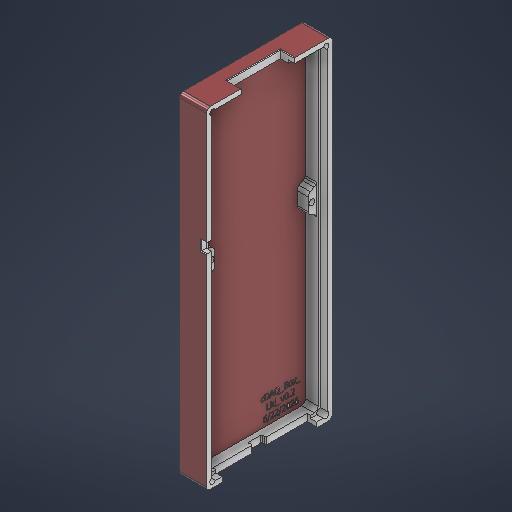
# Autodesk Inventor part: cDAQ_Box_Lid_v0.2
Saved by Autodesk Inventor 2027 (Build 310192000, 192)
## iProperties
Created: 2026-05-08
Part Number: cDAQ_Box_Lid_v0.2
Material: Generic
Document SubType Name: Modeling
Designer: giese
Density: 1 g/cm^3
Appearance: Default
Author: giese
Autodesk Inventor part; units mm, degrees
(part 1 of 2)
ref_plane "YZ Plane" through (0, 0, 0) normal (1, 0, 0) x (0, 1, 0)
ref_plane "XZ Plane" through (0, 0, 0) normal (0, 1, 0) x (-1, 0, 0)
ref_plane "XY Plane" through (0, 0, 0) normal (0, 0, 1) x (1, 0, 0)
sketch "Sketch1" plane through (0, 0, 0) normal (1, 0, 0) x (0, 1, 0)
  line L0 (50.7569, 48.4212) -> (-216.9591, 48.4212)
  line L1 (-216.9591, 48.4212) -> (-216.9591, -53.1788)
  line L2 (-216.9591, -53.1788) -> (50.7569, -53.1788)
  line L3 (50.7569, -53.1788) -> (50.7569, 48.4212)
  point P0 (0, 0)
  dimension "d0" = 101.6
  dimension "d1" = 267.716
  constraints: 8 end point, 2 parallel, 1 horizontal, 1 perpendicular
  measures "d0" distance of L2.end L0.start
  measures "d1" distance of L0.start L0.end
extrude "Extrusion1" add sketch "Sketch1" along normal blind 21.59
sketch "Sketch2" plane through (21.59, 0, 0) normal (1, 0, 0) x (0, 0, -1)
  line L0 (-42.0712, 44.4069) -> (46.8288, 44.4069)
  line L1 (46.8288, 44.4069) -> (46.8288, -210.6091)
  line L2 (46.8288, -210.6091) -> (-42.0712, -210.6091)
  line L3 (-42.0712, -210.6091) -> (-42.0712, 44.4069)
  line L4 (-48.4212, 50.7569) -> (-48.4212, -216.9591) projected
  line L5 (-48.4212, -216.9591) -> (53.1788, -216.9591) projected
  point P0 (0, 0)
  dimension "d4" = 88.9
  dimension "d5" = 255.016
  dimension "d6" = 6.35
  dimension "d7" = 6.35
  constraints: 8 end point, 2 parallel, 1 horizontal, 1 perpendicular
  measures "d4" distance of L0.start L0.end
  measures "d5" distance of L0.end L1.end
  measures "d6" distance between parallel lines of L4 L3
  measures "d7" distance between parallel lines of L5 L2
extrude "Extrusion2" cut sketch "Sketch2" against normal blind 15.24
sketch "Sketch3" plane through (0, 0, 0) normal (-1, 0, 0) x (0, 0, 1)
  circle A0 centre (-30.3188, 7.3229) radius 2
  line L0 (-53.1788, -216.9591) -> (-53.1788, 50.7569) projected
  line L1 (-53.1788, 50.7569) -> (48.4212, 50.7569) projected
  circle A1 centre (-11.82, 7.3229) radius 2
  circle A2 centre (6.6789, 7.3229) radius 2
  point P0 (0, 0)
  dimension "d10" = 22.86
  dimension "d11" = 43.434
  dimension "d12" = 43.434
  dimension "d13" = 18.4988
  dimension "d14" = 4
  dimension "d15" = 4
  dimension "d16" = 43.434
  dimension "d17" = 18.4988
  dimension "d18" = 36.9976
  dimension "d21" = 4
  constraints: 3 centre point
  measures "d10" distance from line of L0 A0.centre
  measures "d11" distance from line of L1 A0.centre
  measures "d12" distance from line of L1 A1.centre
  measures "d13" distance of A0.centre A1.centre
  measures "d14" diameter of A1
  measures "d15" diameter of A2
  measures "d16" distance from line of L1 A2.centre
  measures "d17" distance of A1.centre A2.centre
  measures "d18" distance of A0.centre A2.centre
  measures "d21" diameter of A0
extrude "Extrusion3" [suppressed]
sketch "Sketch6" plane through (0, 50.7569, 48.4212) normal (0, 1, 0) x (1, 0, 0)
  line L0 (21.59, 6.35) -> (21.59, 95.25) projected
  line L1 (10.16, 27.94) -> (21.59, 27.94)
  line L2 (21.59, 27.94) -> (21.59, 71.12)
  line L3 (21.59, 71.12) -> (10.16, 71.12)
  line L4 (10.16, 71.12) -> (10.16, 27.94)
  line L5 (0, 101.6) -> (21.59, 101.6) projected
  point P0 (0, 48.4212)
  point P1 (15.875, 71.12)
  point P2 (15.875, 27.94)
  dimension "d30" = 11.43
  dimension "d31" = 43.18
  dimension "d32" = 30.48
  constraints: 8 end point, 2 midpoint, 2 parallel, 1 horizontal, 1 perpendicular, 1 point on line
  measures "d30" distance between parallel lines of L0 L4
  measures "d31" distance of point (15.875, 71.12) point (15.875, 27.94)
  measures "d32" distance between parallel lines of L5 L3
extrude "Extrusion5" cut sketch "Sketch6" against normal blind 6.35
fillet "Fillet1" radius 3.175 4 edges at (10.795, 50.7569, -53.1788) (10.795, 50.7569, 48.4212) (10.795, -216.9591, 48.4212) (10.795, -216.9591, -53.1788)
sketch "Sketch7" plane through (21.59, 0, 0) normal (1, 0, 0) x (0, 0, -1)
  line L0 (-42.0712, -210.6091) -> (-42.0712, 44.4069) projected
  line L1 (-42.0712, 44.4069) -> (-42.3252, 44.4069)
  line L2 (-42.3252, 46.6929) -> (-44.2302, 46.6929)
  line L3 (-44.2302, 46.6929) -> (-44.2302, 51.0109)
  line L4 (-42.0712, -190.1621) -> (-42.0712, -210.6091)
  line L5 (46.8288, -210.6091) -> (-42.0712, -210.6091) projected
  line L6 (-40.4202, -212.8951) -> (-44.2302, -212.8951)
  line L7 (-44.2302, -212.8951) -> (-44.2302, -190.1621)
  line L8 (46.8288, 44.4069) -> (46.8288, -210.6091) projected
  line L9 (46.8288, -192.7021) -> (46.8288, -210.6091)
  line L10 (46.8288, -210.6091) -> (43.9078, -210.6091)
  line L11 (46.8288, -210.6091) -> (46.8288, -192.7021)
  line L12 (48.9878, -192.7021) -> (48.9878, -212.8951)
  line L13 (48.9878, -212.8951) -> (43.9078, -212.8951)
  line L14 (-42.0712, 44.4069) -> (46.8288, 44.4069) projected
  line L15 (42.0028, 44.4069) -> (46.8288, 44.4069)
  line L16 (48.9878, 48.4709) -> (48.9878, 46.6929)
  line L17 (48.9878, 46.6929) -> (42.0028, 46.6929)
  line L18 (-42.3252, 46.6929) -> (42.0028, 46.6929)
  line L19 (42.0028, 44.4069) -> (-42.3252, 44.4069)
  line L20 (48.9878, 48.4709) -> (48.9878, -192.7021)
  line L21 (44.2888, -195.2421) -> (44.2888, 44.4069)
  line L22 (43.9078, -210.6091) -> (-40.4202, -210.6091)
  line L23 (-40.4202, -212.8951) -> (43.9078, -212.8951)
  line L24 (-44.2302, -190.1621) -> (-44.2302, 51.0109)
  line L25 (-42.0712, 44.4069) -> (-42.0712, -190.1621)
  point P0 (0, 0)
  point P1 (-42.0712, 51.0109)
  point P2 (-44.2302, 48.9789)
  point P3 (46.8288, 48.4709)
  point P4 (48.9878, 46.6929)
  point P5 (-44.2302, 46.6929)
  dimension "d34" = 2.286
  dimension "d35" = 2.159
  dimension "d38" = 2.159
  dimension "d39" = 2.286
  dimension "d42" = 2.286
  dimension "d43" = 2.159
  dimension "d46" = 2.286
  dimension "d47" = 2.159
  constraints: 44 end point, 9 point on line, 4 parallel, 4 perpendicular, 2 collinear, 2 horizontal, 2 vertical
  measures "d34" distance between parallel lines of L2 L1
  measures "d35" distance between parallel lines of L0 L3
  measures "d38" distance between parallel lines of L7 L0
  measures "d39" distance between parallel lines of L5 L6
  measures "d42" distance between parallel lines of L5 L13
  measures "d43" distance between parallel lines of L8 L12
  measures "d46" distance between parallel lines of L14 L17
  measures "d47" distance between parallel lines of L8 L16
extrude "Extrusion6" cut sketch "Sketch7" against normal blind 5 contours L0 L14 L8 L5 | L18 L17 L20 L12 L13 L23 L6 L7 L24 L2
fillet "Fillet2" radius 3.175 8 edges at (19.09, 46.6929, 44.2302) (11.47, 44.4069, 42.0712) (19.09, 46.6929, -48.9878) (11.47, 44.4069, -46.8288) (11.47, -210.6091, 42.0712) (19.09, -212.8951, 44.2302) (11.47, -210.6091, -46.8288) (19.09, -212.8951, -48.9878)
sketch "Sketch11" plane through (16.59, 0, 0) normal (1, 0, 0) x (0, 0, -1)
  circle A0 centre (48.0988, 45.6769) radius 2.4005
  line L0 (50.0038, 50.7569) -> (22.6988, 50.7569) projected
  line L1 (53.1788, -213.7841) -> (53.1788, 47.5819) projected
  arc A1 (46.9238, 45.7719) -> (43.7488, 48.9469) centre (43.7488, 45.7719) ccw projected
  circle A2 centre (-43.3412, 45.6769) radius 2.4005
  line L2 (-48.4212, 47.5819) -> (-48.4212, -213.7841) projected
  line L3 (-20.4812, 50.7569) -> (-45.2462, 50.7569) projected
  circle A3 centre (48.0988, -211.8791) radius 2.4005
  line L4 (-45.2462, -216.9591) -> (50.0038, -216.9591) projected
  circle A4 centre (-43.3412, -211.8791) radius 2.4005
  circle A5 centre (43.0188, -63.5431) radius 2.4005
  circle A6 centre (-38.2612, -63.5431) radius 2.4005
  point P0 (0, 0)
  point P1 (45.9939, 48.017)
  point P2 (48.5528, -43.2993)
  point P3 (45.3778, -46.4743)
  point P4 (-30.4007, -42.8803)
  point P5 (-33.5757, -46.0553)
  dimension "d58" = 4.801
  dimension "d59" = 5.08
  dimension "d60" = 5.08
  dimension "d61" = 4.801
  dimension "d62" = 4.801
  dimension "d63" = 5.08
  dimension "d64" = 5.08
  dimension "d65" = 4.801
  dimension "d66" = 5.08
  dimension "d67" = 5.08
  dimension "d76" = 5.08
  dimension "d77" = 5.08
  dimension "d114" = 4.801
  dimension "d115" = 114.3
  dimension "d116" = 10.16
  dimension "d117" = 4.801
  dimension "d118" = 114.3
  dimension "d119" = 10.16
  constraints: 6 centre point, 1 point on circle
  measures "d58" diameter of A0
  measures "d59" distance from line of L2 A2.centre
  measures "d60" distance from line of L3 A2.centre
  measures "d61" diameter of A2
  measures "d62" diameter of A3
  measures "d63" distance from line of L1 A3.centre
  measures "d64" distance from line of L4 A3.centre
  measures "d65" diameter of A4
  measures "d66" distance from line of L2 A4.centre
  measures "d67" distance from line of L4 A4.centre
  measures "d76" distance from line of L1 A0.centre
  measures "d77" distance from line of L0 A0.centre
  measures "d114" diameter of A5
  measures "d115" distance from line of A5.centre L0
  measures "d116" distance from line of L1 A5.centre
  measures "d117" diameter of A6
  measures "d118" distance from line of A6.centre L3
  measures "d119" distance from line of L2 A6.centre
extrude "Extrusion8" cut sketch "Sketch11" along normal blind 5.08 and the other way blind 17.78
sketch "Sketch13" plane through (6.35, 0, 0) normal (1, 0, 0) x (0, 0, -1)
  line L0 (14.3842, -187.8124) -> (39.44, -187.8124) construction
  line L1 (39.44, -187.8124) -> (39.44, -196.6766) construction
  line L2 (39.44, -196.6766) -> (14.3842, -196.6766) construction
  line L3 (14.3842, -196.6766) -> (14.3842, -187.8124) construction
  spline S0 degree 2 poles (12.407, -192.5585) (12.0513, -192.5585) (11.4622, -192.3399) (11.251, -192.1176) knots 0 0 0 1 2 2 2
  spline S1 degree 2 poles (11.251, -192.1176) (11.0398, -191.899) (10.8064, -191.2247) (10.8064, -190.7727) knots 0 0 0 1 2 2 2
  spline S2 degree 2 poles (10.8064, -190.7727) (10.8064, -190.3207) (11.0472, -189.6612) (11.251, -189.4389) knots 0 0 0 1 2 2 2
  spline S3 degree 2 poles (11.251, -189.4389) (11.4548, -189.2129) (12.0587, -188.972) (12.407, -188.972) knots 0 0 0 1 2 2 2
  spline S4 degree 2 poles (12.407, -188.972) (12.6885, -188.972) (13.2146, -189.1313) (13.4184, -189.2351) knots 0 0 0 1 2 2 2
  line L4 (13.4184, -189.2351) -> (13.4184, -189.8835)
  line L5 (13.4184, -189.8835) -> (13.3851, -189.8835)
  spline S5 degree 2 poles (13.3851, -189.8835) (13.3221, -189.8316) (13.1294, -189.6982) (12.9923, -189.6278) knots 0 0 0 1 2 2 2
  spline S6 degree 2 poles (12.9923, -189.6278) (12.8701, -189.5685) (12.544, -189.4759) (12.3958, -189.4759) knots 0 0 0 1 2 2 2
  spline S7 degree 2 poles (12.3958, -189.4759) (11.9475, -189.4759) (11.4029, -190.1539) (11.4029, -190.7727) knots 0 0 0 1 2 2 2
  spline S8 degree 2 poles (11.4029, -190.7727) (11.4029, -191.3766) (11.929, -192.0546) (12.3958, -192.0546) knots 0 0 0 1 2 2 2
  spline S9 degree 2 poles (12.3958, -192.0546) (12.6774, -192.0546) (13.1887, -191.8212) (13.3851, -191.6396) knots 0 0 0 1 2 2 2
  line L6 (13.3851, -191.6396) -> (13.4184, -191.6396)
  line L7 (13.4184, -191.6396) -> (13.4184, -192.288)
  spline S10 degree 2 poles (13.4184, -192.288) (13.3332, -192.3288) (13.0739, -192.4436) (12.9701, -192.4696) knots 0 0 0 1 2 2 2
  spline S11 degree 2 poles (12.9701, -192.4696) (12.8219, -192.514) (12.5885, -192.5585) (12.407, -192.5585) knots 0 0 0 1 2 2 2
  spline S12 degree 2 poles (17.594, -190.1984) (17.594, -190.8245) (17.0864, -191.8323) (16.6603, -192.1139) knots 0 0 0 1 2 2 2
  spline S13 degree 2 poles (16.6603, -192.1139) (16.3121, -192.3325) (15.597, -192.4807) (15.0412, -192.4807) knots 0 0 0 1 2 2 2
  line L8 (15.0412, -192.4807) -> (13.989, -192.4807)
  line L9 (13.989, -192.4807) -> (13.989, -187.9087)
  line L10 (13.989, -187.9087) -> (15.0301, -187.9087)
  spline S14 degree 2 poles (15.0301, -187.9087) (15.6748, -187.9087) (16.4084, -188.1013) (16.6677, -188.2718) knots 0 0 0 1 2 2 2
  spline S15 degree 2 poles (16.6677, -188.2718) (17.1086, -188.5645) (17.594, -189.5315) (17.594, -190.1984) knots 0 0 0 1 2 2 2
  spline S16 degree 2 poles (16.9604, -190.191) (16.9604, -189.6649) (16.6122, -188.9202) (16.2676, -188.709) knots 0 0 0 1 2 2 2
  spline S17 degree 2 poles (16.2676, -188.709) (16.0231, -188.5645) (15.471, -188.4348) (15.0598, -188.4348) knots 0 0 0 1 2 2 2
  line L11 (15.0598, -188.4348) -> (14.5966, -188.4348)
  line L12 (14.5966, -188.4348) -> (14.5966, -191.9546)
  line L13 (14.5966, -191.9546) -> (15.0598, -191.9546)
  spline S18 degree 2 poles (15.0598, -191.9546) (15.4636, -191.9546) (16.0749, -191.8249) (16.3232, -191.6508) knots 0 0 0 1 2 2 2
  spline S19 degree 2 poles (16.3232, -191.6508) (16.6418, -191.4359) (16.9604, -190.7245) (16.9604, -190.191) knots 0 0 0 1 2 2 2
  line L14 (17.7607, -192.4807) -> (19.302, -187.9087)
  line L15 (19.302, -187.9087) -> (20.0504, -187.9087)
  line L16 (20.0504, -187.9087) -> (21.5917, -192.4807)
  line L17 (21.5917, -192.4807) -> (20.9507, -192.4807)
  line L18 (20.9507, -192.4807) -> (20.5358, -191.2025)
  line L19 (20.5358, -191.2025) -> (18.7907, -191.2025)
  line L20 (18.7907, -191.2025) -> (18.3757, -192.4807)
  line L21 (18.3757, -192.4807) -> (17.7607, -192.4807)
  line L22 (20.3691, -190.6838) -> (19.6614, -188.5311)
  line L23 (19.6614, -188.5311) -> (18.9574, -190.6838)
  line L24 (18.9574, -190.6838) -> (20.3691, -190.6838)
  spline S20 degree 2 poles (25.8228, -193.5996) (25.6561, -193.6404) (25.293, -193.6848) (25.1115, -193.6848) knots 0 0 0 1 2 2 2
  spline S21 degree 2 poles (25.1115, -193.6848) (24.5965, -193.6848) (23.9555, -193.1105) (23.9259, -192.577) knots 0 0 0 1 2 2 2
  spline S22 degree 2 poles (23.9259, -192.577) (23.8851, -192.577) (23.8147, -192.577) (23.7851, -192.577) knots 0 0 0 1 2 2 2
  spline S23 degree 2 poles (23.7851, -192.577) (23.322, -192.577) (22.5772, -192.2621) (22.3105, -191.9546) knots 0 0 0 1 2 2 2
  spline S24 degree 2 poles (22.3105, -191.9546) (22.0474, -191.6508) (21.7658, -190.7616) (21.7658, -190.1984) knots 0 0 0 1 2 2 2
  spline S25 degree 2 poles (21.7658, -190.1984) (21.7658, -189.6204) (22.0511, -188.746) (22.3142, -188.4348) knots 0 0 0 1 2 2 2
  spline S26 degree 2 poles (22.3142, -188.4348) (22.581, -188.1273) (23.3257, -187.8124) (23.7851, -187.8124) knots 0 0 0 1 2 2 2
  spline S27 degree 2 poles (23.7851, -187.8124) (24.2519, -187.8124) (25.0003, -188.1384) (25.2597, -188.4348) knots 0 0 0 1 2 2 2
  spline S28 degree 2 poles (25.2597, -188.4348) (25.519, -188.7349) (25.808, -189.6278) (25.808, -190.1984) knots 0 0 0 1 2 2 2
  spline S29 degree 2 poles (25.808, -190.1984) (25.808, -191.0876) (25.1152, -192.2436) (24.5113, -192.4473) knots 0 0 0 1 2 2 2
  spline S30 degree 2 poles (24.5113, -192.4473) (24.5261, -192.6178) (24.615, -192.8919) (24.6854, -192.9698) knots 0 0 0 1 2 2 2
  spline S31 degree 2 poles (24.6854, -192.9698) (24.7706, -193.0661) (25.004, -193.155) (25.2115, -193.155) knots 0 0 0 1 2 2 2
  spline S32 degree 2 poles (25.2115, -193.155) (25.3338, -193.155) (25.6672, -193.0772) (25.7413, -193.0476) knots 0 0 0 1 2 2 2
  line L25 (25.7413, -193.0476) -> (25.8228, -193.0476)
  line L26 (25.8228, -193.0476) -> (25.8228, -193.5996)
  spline S33 degree 2 poles (25.1745, -190.1984) (25.1745, -189.7427) (24.9781, -189.0424) (24.8003, -188.8127) knots 0 0 0 1 2 2 2
  spline S34 degree 2 poles (24.8003, -188.8127) (24.6187, -188.5756) (24.1074, -188.3385) (23.7888, -188.3385) knots 0 0 0 1 2 2 2
  spline S35 degree 2 poles (23.7888, -188.3385) (23.459, -188.3385) (22.9626, -188.5682) (22.7736, -188.8127) knots 0 0 0 1 2 2 2
  spline S36 degree 2 poles (22.7736, -188.8127) (22.5921, -189.0461) (22.3994, -189.7538) (22.3994, -190.1984) knots 0 0 0 1 2 2 2
  spline S37 degree 2 poles (22.3994, -190.1984) (22.3994, -191.0987) (23.1552, -192.0583) (23.7888, -192.0583) knots 0 0 0 1 2 2 2
  spline S38 degree 2 poles (23.7888, -192.0583) (24.4223, -192.0583) (25.1745, -191.0987) (25.1745, -190.1984) knots 0 0 0 1 2 2 2
  line L27 (29.4908, -193.3995) -> (25.9636, -193.3995)
  line L28 (25.9636, -193.3995) -> (25.9636, -193.0031)
  line L29 (25.9636, -193.0031) -> (29.4908, -193.0031)
  line L30 (29.4908, -193.0031) -> (29.4908, -193.3995)
  spline S39 degree 2 poles (33.0069, -191.0765) (33.0069, -191.4173) (32.7475, -191.9398) (32.5326, -192.1102) knots 0 0 0 1 2 2 2
  spline S40 degree 2 poles (32.5326, -192.1102) (32.2733, -192.3103) (31.6842, -192.4807) (31.2174, -192.4807) knots 0 0 0 1 2 2 2
  line L31 (31.2174, -192.4807) -> (29.9058, -192.4807)
  line L32 (29.9058, -192.4807) -> (29.9058, -187.9087)
  line L33 (29.9058, -187.9087) -> (31.1173, -187.9087)
  spline S41 degree 2 poles (31.1173, -187.9087) (31.6064, -187.9087) (32.0955, -187.9717) (32.3178, -188.0939) knots 0 0 0 1 2 2 2
  spline S42 degree 2 poles (32.3178, -188.0939) (32.566, -188.2236) (32.792, -188.6497) (32.792, -188.9387) knots 0 0 0 1 2 2 2
  spline S43 degree 2 poles (32.792, -188.9387) (32.792, -189.261) (32.4511, -189.7723) (32.151, -189.9168) knots 0 0 0 1 2 2 2
  line L34 (32.151, -189.9168) -> (32.151, -189.939)
  spline S44 degree 2 poles (32.151, -189.939) (32.5586, -190.0502) (33.0069, -190.6393) (33.0069, -191.0765) knots 0 0 0 1 2 2 2
  spline S45 degree 2 poles (32.3733, -191.1024) (32.3733, -190.8431) (32.2251, -190.5096) (32.0028, -190.3911) knots 0 0 0 1 2 2 2
  spline S46 degree 2 poles (32.0028, -190.3911) (31.8583, -190.317) (31.5175, -190.2725) (31.2025, -190.2725) knots 0 0 0 1 2 2 2
  line L35 (31.2025, -190.2725) -> (30.5134, -190.2725)
  line L36 (30.5134, -190.2725) -> (30.5134, -191.962)
  line L37 (30.5134, -191.962) -> (31.0062, -191.962)
  spline S47 degree 2 poles (31.0062, -191.962) (31.4063, -191.962) (31.8657, -191.8879) (32.0436, -191.7693) knots 0 0 0 1 2 2 2
  spline S48 degree 2 poles (32.0436, -191.7693) (32.214, -191.6471) (32.3733, -191.3432) (32.3733, -191.1024) knots 0 0 0 1 2 2 2
  spline S49 degree 2 poles (32.1584, -189.0239) (32.1584, -188.8609) (32.0473, -188.6163) (31.925, -188.546) knots 0 0 0 1 2 2 2
  spline S50 degree 2 poles (31.925, -188.546) (31.7768, -188.4644) (31.4174, -188.4274) (31.0951, -188.4274) knots 0 0 0 1 2 2 2
  line L38 (31.0951, -188.4274) -> (30.5134, -188.4274)
  line L39 (30.5134, -188.4274) -> (30.5134, -189.7649)
  line L40 (30.5134, -189.7649) -> (31.2025, -189.7649)
  spline S51 degree 2 poles (31.2025, -189.7649) (31.4878, -189.7649) (31.7583, -189.7056) (31.9028, -189.613) knots 0 0 0 1 2 2 2
  spline S52 degree 2 poles (31.9028, -189.613) (32.0436, -189.5241) (32.1584, -189.2388) (32.1584, -189.0239) knots 0 0 0 1 2 2 2
  spline S53 degree 2 poles (36.3859, -190.7653) (36.3859, -191.6322) (35.5522, -192.577) (34.8557, -192.577) knots 0 0 0 1 2 2 2
  spline S54 degree 2 poles (34.8557, -192.577) (34.1406, -192.577) (33.3218, -191.6026) (33.3218, -190.7653) knots 0 0 0 1 2 2 2
  spline S55 degree 2 poles (33.3218, -190.7653) (33.3218, -189.9057) (34.1666, -188.9535) (34.8557, -188.9535) knots 0 0 0 1 2 2 2
  spline S56 degree 2 poles (34.8557, -188.9535) (35.5522, -188.9535) (36.3859, -189.902) (36.3859, -190.7653) knots 0 0 0 1 2 2 2
  spline S57 degree 2 poles (35.7894, -190.7653) (35.7894, -190.0984) (35.304, -189.45) (34.8557, -189.45) knots 0 0 0 1 2 2 2
  spline S58 degree 2 poles (34.8557, -189.45) (34.4074, -189.45) (33.9183, -190.0984) (33.9183, -190.7653) knots 0 0 0 1 2 2 2
  spline S59 degree 2 poles (33.9183, -190.7653) (33.9183, -191.4136) (34.4074, -192.0805) (34.8557, -192.0805) knots 0 0 0 1 2 2 2
  spline S60 degree 2 poles (34.8557, -192.0805) (35.3003, -192.0805) (35.7894, -191.4248) (35.7894, -190.7653) knots 0 0 0 1 2 2 2
  line L41 (39.6426, -192.4807) -> (38.9349, -192.4807)
  line L42 (38.9349, -192.4807) -> (38.1013, -191.1913)
  line L43 (38.1013, -191.1913) -> (37.2454, -192.4807)
  line L44 (37.2454, -192.4807) -> (36.5896, -192.4807)
  line L45 (36.5896, -192.4807) -> (37.779, -190.7801)
  line L46 (37.779, -190.7801) -> (36.6008, -189.0498)
  line L47 (36.6008, -189.0498) -> (37.3084, -189.0498)
  line L48 (37.3084, -189.0498) -> (38.1383, -190.3281)
  line L49 (38.1383, -190.3281) -> (38.9868, -189.0498)
  line L50 (38.9868, -189.0498) -> (39.6426, -189.0498)
  line L51 (39.6426, -189.0498) -> (38.4607, -190.743)
  line L52 (38.4607, -190.743) -> (39.6426, -192.4807)
  line L53 (43.1512, -193.3995) -> (39.6241, -193.3995)
  line L54 (39.6241, -193.3995) -> (39.6241, -193.0031)
  line L55 (39.6241, -193.0031) -> (43.1512, -193.0031)
  line L56 (43.1512, -193.0031) -> (43.1512, -193.3995)
  line L57 (18.3406, -200.0084) -> (15.6915, -200.0084)
  line L58 (15.6915, -200.0084) -> (15.6915, -195.4364)
  line L59 (15.6915, -195.4364) -> (16.2991, -195.4364)
  line L60 (16.2991, -195.4364) -> (16.2991, -199.4674)
  line L61 (16.2991, -199.4674) -> (18.3406, -199.4674)
  line L62 (18.3406, -199.4674) -> (18.3406, -200.0084)
  line L63 (19.3631, -200.0084) -> (18.7852, -200.0084)
  line L64 (18.7852, -200.0084) -> (18.7852, -196.5775)
  line L65 (18.7852, -196.5775) -> (19.3631, -196.5775)
  line L66 (19.3631, -196.5775) -> (19.3631, -200.0084)
  line L67 (19.4039, -196.0069) -> (18.7481, -196.0069)
  line L68 (18.7481, -196.0069) -> (18.7481, -195.4067)
  line L69 (18.7481, -195.4067) -> (19.4039, -195.4067)
  line L70 (19.4039, -195.4067) -> (19.4039, -196.0069)
  line L71 (22.8496, -200.0084) -> (22.2716, -200.0084)
  line L72 (22.2716, -200.0084) -> (22.2716, -199.6601)
  spline S61 degree 2 poles (22.2716, -199.6601) (22.1382, -199.7712) (21.9418, -199.9194) (21.8085, -199.9824) knots 0 0 0 1 2 2 2
  spline S62 degree 2 poles (21.8085, -199.9824) (21.6862, -200.0417) (21.4231, -200.1047) (21.249, -200.1047) knots 0 0 0 1 2 2 2
  spline S63 degree 2 poles (21.249, -200.1047) (20.9674, -200.1047) (20.4932, -199.8713) (20.3264, -199.6453) knots 0 0 0 1 2 2 2
  spline S64 degree 2 poles (20.3264, -199.6453) (20.1597, -199.4193) (19.9745, -198.7524) (19.9745, -198.3189) knots 0 0 0 1 2 2 2
  spline S65 degree 2 poles (19.9745, -198.3189) (19.9745, -197.8669) (20.2079, -197.2074) (20.4117, -196.9591) knots 0 0 0 1 2 2 2
  spline S66 degree 2 poles (20.4117, -196.9591) (20.6006, -196.7368) (21.1304, -196.4812) (21.4231, -196.4812) knots 0 0 0 1 2 2 2
  spline S67 degree 2 poles (21.4231, -196.4812) (21.6788, -196.4812) (22.0604, -196.596) (22.2716, -196.7146) knots 0 0 0 1 2 2 2
  line L73 (22.2716, -196.7146) -> (22.2716, -195.2326)
  line L74 (22.2716, -195.2326) -> (22.8496, -195.2326)
  line L75 (22.8496, -195.2326) -> (22.8496, -200.0084)
  line L76 (22.2716, -199.1747) -> (22.2716, -197.1925)
  spline S68 degree 2 poles (22.2716, -197.1925) (22.0567, -197.0888) (21.7158, -197.011) (21.5195, -197.011) knots 0 0 0 1 2 2 2
  spline S69 degree 2 poles (21.5195, -197.011) (21.0749, -197.011) (20.571, -197.6779) (20.571, -198.3078) knots 0 0 0 1 2 2 2
  spline S70 degree 2 poles (20.571, -198.3078) (20.571, -198.9154) (20.9563, -199.5564) (21.3824, -199.5564) knots 0 0 0 1 2 2 2
  spline S71 degree 2 poles (21.3824, -199.5564) (21.6084, -199.5564) (22.0678, -199.3489) (22.2716, -199.1747) knots 0 0 0 1 2 2 2
  line L77 (26.7473, -200.9272) -> (23.2201, -200.9272)
  line L78 (23.2201, -200.9272) -> (23.2201, -200.5308)
  line L79 (23.2201, -200.5308) -> (26.7473, -200.5308)
  line L80 (26.7473, -200.5308) -> (26.7473, -200.9272)
  line L81 (29.8113, -196.5775) -> (28.5183, -200.0084)
  line L82 (28.5183, -200.0084) -> (27.9995, -200.0084)
  line L83 (27.9995, -200.0084) -> (26.7176, -196.5775)
  line L84 (26.7176, -196.5775) -> (27.3438, -196.5775)
  line L85 (27.3438, -196.5775) -> (28.2811, -199.2192)
  line L86 (28.2811, -199.2192) -> (29.2111, -196.5775)
  line L87 (29.2111, -196.5775) -> (29.8113, -196.5775)
  spline S72 degree 2 poles (33.0087, -197.7224) (33.0087, -198.9524) (32.2937, -200.1047) (31.549, -200.1047) knots 0 0 0 1 2 2 2
  spline S73 degree 2 poles (31.549, -200.1047) (30.7931, -200.1047) (30.0855, -198.9302) (30.0855, -197.7261) knots 0 0 0 1 2 2 2
  spline S74 degree 2 poles (30.0855, -197.7261) (30.0855, -196.4886) (30.8005, -195.3437) (31.549, -195.3437) knots 0 0 0 1 2 2 2
  spline S75 degree 2 poles (31.549, -195.3437) (32.3011, -195.3437) (33.0087, -196.5293) (33.0087, -197.7224) knots 0 0 0 1 2 2 2
  spline S76 degree 2 poles (32.2233, -199.1155) (32.3122, -198.8894) (32.3863, -198.1929) (32.3863, -197.7224) knots 0 0 0 1 2 2 2
  spline S77 degree 2 poles (32.3863, -197.7224) (32.3863, -197.2518) (32.3122, -196.559) (32.2196, -196.3256) knots 0 0 0 1 2 2 2
  spline S78 degree 2 poles (32.2196, -196.3256) (32.1269, -196.0922) (31.8046, -195.8513) (31.549, -195.8513) knots 0 0 0 1 2 2 2
  spline S79 degree 2 poles (31.549, -195.8513) (31.2933, -195.8513) (30.9636, -196.0922) (30.8672, -196.333) knots 0 0 0 1 2 2 2
  spline S80 degree 2 poles (30.8672, -196.333) (30.7746, -196.5664) (30.7079, -197.2778) (30.7079, -197.7261) knots 0 0 0 1 2 2 2
  spline S81 degree 2 poles (30.7079, -197.7261) (30.7079, -198.2077) (30.7672, -198.8524) (30.8635, -199.1043) knots 0 0 0 1 2 2 2
  spline S82 degree 2 poles (30.8635, -199.1043) (30.9525, -199.3415) (31.2822, -199.5971) (31.549, -199.5971) knots 0 0 0 1 2 2 2
  spline S83 degree 2 poles (31.549, -199.5971) (31.8009, -199.5971) (32.1307, -199.3563) (32.2233, -199.1155) knots 0 0 0 1 2 2 2
  line L88 (34.576, -200.0084) -> (33.8424, -200.0084)
  line L89 (33.8424, -200.0084) -> (33.8424, -199.134)
  line L90 (33.8424, -199.134) -> (34.576, -199.134)
  line L91 (34.576, -199.134) -> (34.576, -200.0084)
  line L92 (38.318, -200.0084) -> (35.4985, -200.0084)
  line L93 (35.4985, -200.0084) -> (35.4985, -199.36)
  spline S84 degree 2 poles (35.4985, -199.36) (35.8023, -199.0747) (36.3433, -198.5449) (36.6026, -198.2596) knots 0 0 0 1 2 2 2
  spline S85 degree 2 poles (36.6026, -198.2596) (37.125, -197.6853) (37.5066, -196.9962) (37.5066, -196.6294) knots 0 0 0 1 2 2 2
  spline S86 degree 2 poles (37.5066, -196.6294) (37.5066, -196.4367) (37.3881, -196.1477) (37.2806, -196.0551) knots 0 0 0 1 2 2 2
  spline S87 degree 2 poles (37.2806, -196.0551) (37.1732, -195.9625) (36.8916, -195.8699) (36.7212, -195.8699) knots 0 0 0 1 2 2 2
  spline S88 degree 2 poles (36.7212, -195.8699) (36.5582, -195.8699) (36.2247, -195.9514) (36.0728, -196.0143) knots 0 0 0 1 2 2 2
  spline S89 degree 2 poles (36.0728, -196.0143) (35.9431, -196.0662) (35.7023, -196.2144) (35.6282, -196.2663) knots 0 0 0 1 2 2 2
  line L94 (35.6282, -196.2663) -> (35.5948, -196.2663)
  line L95 (35.5948, -196.2663) -> (35.5948, -195.6142)
  spline S90 degree 2 poles (35.5948, -195.6142) (35.7838, -195.5216) (36.4618, -195.34) (36.7656, -195.34) knots 0 0 0 1 2 2 2
  spline S91 degree 2 poles (36.7656, -195.34) (37.4066, -195.34) (38.1291, -196.0181) (38.1291, -196.596) knots 0 0 0 1 2 2 2
  spline S92 degree 2 poles (38.1291, -196.596) (38.1291, -196.8665) (38.0031, -197.3185) (37.892, -197.5112) knots 0 0 0 1 2 2 2
  spline S93 degree 2 poles (37.892, -197.5112) (37.7808, -197.7113) (37.4585, -198.104) (37.2806, -198.2929) knots 0 0 0 1 2 2 2
  spline S94 degree 2 poles (37.2806, -198.2929) (36.9916, -198.6079) (36.284, -199.2822) (36.0728, -199.4785) knots 0 0 0 1 2 2 2
  line L96 (36.0728, -199.4785) -> (38.318, -199.4785)
  line L97 (38.318, -199.4785) -> (38.318, -200.0084)
  spline S95 degree 2 poles (15.723, -206.054) (15.723, -206.406) (15.4895, -207.0025) (15.2932, -207.2026) knots 0 0 0 1 2 2 2
  spline S96 degree 2 poles (15.2932, -207.2026) (15.0894, -207.4138) (14.5781, -207.6324) (14.2706, -207.6324) knots 0 0 0 1 2 2 2
  spline S97 degree 2 poles (14.2706, -207.6324) (13.9631, -207.6324) (13.4555, -207.4249) (13.2628, -207.2174) knots 0 0 0 1 2 2 2
  spline S98 degree 2 poles (13.2628, -207.2174) (13.0257, -206.9692) (12.7589, -206.1355) (12.7589, -205.5279) knots 0 0 0 1 2 2 2
  spline S99 degree 2 poles (12.7589, -205.5279) (12.7589, -204.9314) (13.0035, -203.9718) (13.2591, -203.6161) knots 0 0 0 1 2 2 2
  spline S100 degree 2 poles (13.2591, -203.6161) (13.5073, -203.2679) (14.2928, -202.8788) (14.8078, -202.8788) knots 0 0 0 1 2 2 2
  spline S101 degree 2 poles (14.8078, -202.8788) (14.9597, -202.8788) (15.2265, -202.9085) (15.3265, -202.9418) knots 0 0 0 1 2 2 2
  line L98 (15.3265, -202.9418) -> (15.3265, -203.5309)
  line L99 (15.3265, -203.5309) -> (15.3006, -203.5309)
  spline S102 degree 2 poles (15.3006, -203.5309) (15.2154, -203.4865) (14.9041, -203.4086) (14.7263, -203.4086) knots 0 0 0 1 2 2 2
  spline S103 degree 2 poles (14.7263, -203.4086) (14.1557, -203.4086) (13.4555, -204.1793) (13.3888, -204.9351) knots 0 0 0 1 2 2 2
  spline S104 degree 2 poles (13.3888, -204.9351) (13.6074, -204.7832) (14.0668, -204.6165) (14.341, -204.6165) knots 0 0 0 1 2 2 2
  spline S105 degree 2 poles (14.341, -204.6165) (14.6077, -204.6165) (15.0079, -204.7239) (15.2265, -204.887) knots 0 0 0 1 2 2 2
  spline S106 degree 2 poles (15.2265, -204.887) (15.4784, -205.0759) (15.723, -205.6613) (15.723, -206.054) knots 0 0 0 1 2 2 2
  spline S107 degree 2 poles (15.1005, -206.08) (15.1005, -205.7984) (14.9523, -205.4168) (14.7893, -205.2834) knots 0 0 0 1 2 2 2
  spline S108 degree 2 poles (14.7893, -205.2834) (14.667, -205.1871) (14.3632, -205.1241) (14.2039, -205.1241) knots 0 0 0 1 2 2 2
  spline S109 degree 2 poles (14.2039, -205.1241) (13.989, -205.1241) (13.5852, -205.2537) (13.3888, -205.376) knots 0 0 0 1 2 2 2
  spline S110 degree 2 poles (13.3888, -205.376) (13.3851, -205.4427) (13.3777, -205.5687) (13.3777, -205.665) knots 0 0 0 1 2 2 2
  spline S111 degree 2 poles (13.3777, -205.665) (13.3777, -206.1392) (13.5629, -206.7209) (13.7037, -206.8728) knots 0 0 0 1 2 2 2
  spline S112 degree 2 poles (13.7037, -206.8728) (13.8334, -207.0173) (14.115, -207.1322) (14.2743, -207.1322) knots 0 0 0 1 2 2 2
  spline S113 degree 2 poles (14.2743, -207.1322) (14.6448, -207.1322) (15.1005, -206.6061) (15.1005, -206.08) knots 0 0 0 1 2 2 2
  line L100 (18.1646, -202.7603) -> (16.375, -208.529)
  line L101 (16.375, -208.529) -> (15.8563, -208.529)
  line L102 (15.8563, -208.529) -> (17.6384, -202.7603)
  line L103 (17.6384, -202.7603) -> (18.1646, -202.7603)
  line L104 (21.488, -207.536) -> (18.6684, -207.536)
  line L105 (18.6684, -207.536) -> (18.6684, -206.8877)
  spline S114 degree 2 poles (18.6684, -206.8877) (18.9723, -206.6024) (19.5132, -206.0726) (19.7725, -205.7873) knots 0 0 0 1 2 2 2
  spline S115 degree 2 poles (19.7725, -205.7873) (20.295, -205.213) (20.6766, -204.5239) (20.6766, -204.1571) knots 0 0 0 1 2 2 2
  spline S116 degree 2 poles (20.6766, -204.1571) (20.6766, -203.9644) (20.558, -203.6754) (20.4506, -203.5828) knots 0 0 0 1 2 2 2
  spline S117 degree 2 poles (20.4506, -203.5828) (20.3431, -203.4902) (20.0615, -203.3975) (19.8911, -203.3975) knots 0 0 0 1 2 2 2
  spline S118 degree 2 poles (19.8911, -203.3975) (19.7281, -203.3975) (19.3946, -203.479) (19.2427, -203.542) knots 0 0 0 1 2 2 2
  spline S119 degree 2 poles (19.2427, -203.542) (19.113, -203.5939) (18.8722, -203.7421) (18.7981, -203.794) knots 0 0 0 1 2 2 2
  line L106 (18.7981, -203.794) -> (18.7648, -203.794)
  line L107 (18.7648, -203.794) -> (18.7648, -203.1419)
  spline S120 degree 2 poles (18.7648, -203.1419) (18.9537, -203.0493) (19.6318, -202.8677) (19.9356, -202.8677) knots 0 0 0 1 2 2 2
  spline S121 degree 2 poles (19.9356, -202.8677) (20.5765, -202.8677) (21.299, -203.5457) (21.299, -204.1237) knots 0 0 0 1 2 2 2
  spline S122 degree 2 poles (21.299, -204.1237) (21.299, -204.3942) (21.173, -204.8462) (21.0619, -205.0389) knots 0 0 0 1 2 2 2
  spline S123 degree 2 poles (21.0619, -205.0389) (20.9507, -205.2389) (20.6284, -205.6317) (20.4506, -205.8206) knots 0 0 0 1 2 2 2
  spline S124 degree 2 poles (20.4506, -205.8206) (20.1616, -206.1355) (19.4539, -206.8099) (19.2427, -207.0062) knots 0 0 0 1 2 2 2
  line L108 (19.2427, -207.0062) -> (21.488, -207.0062)
  line L109 (21.488, -207.0062) -> (21.488, -207.536)
  line L110 (24.9188, -207.536) -> (22.0993, -207.536)
  line L111 (22.0993, -207.536) -> (22.0993, -206.8877)
  spline S125 degree 2 poles (22.0993, -206.8877) (22.4031, -206.6024) (22.944, -206.0726) (23.2034, -205.7873) knots 0 0 0 1 2 2 2
  spline S126 degree 2 poles (23.2034, -205.7873) (23.7258, -205.213) (24.1074, -204.5239) (24.1074, -204.1571) knots 0 0 0 1 2 2 2
  spline S127 degree 2 poles (24.1074, -204.1571) (24.1074, -203.9644) (23.9889, -203.6754) (23.8814, -203.5828) knots 0 0 0 1 2 2 2
  spline S128 degree 2 poles (23.8814, -203.5828) (23.774, -203.4902) (23.4924, -203.3975) (23.322, -203.3975) knots 0 0 0 1 2 2 2
  spline S129 degree 2 poles (23.322, -203.3975) (23.1589, -203.3975) (22.8255, -203.479) (22.6736, -203.542) knots 0 0 0 1 2 2 2
  spline S130 degree 2 poles (22.6736, -203.542) (22.5439, -203.5939) (22.3031, -203.7421) (22.229, -203.794) knots 0 0 0 1 2 2 2
  line L112 (22.229, -203.794) -> (22.1956, -203.794)
  line L113 (22.1956, -203.794) -> (22.1956, -203.1419)
  spline S131 degree 2 poles (22.1956, -203.1419) (22.3846, -203.0493) (23.0626, -202.8677) (23.3664, -202.8677) knots 0 0 0 1 2 2 2
  spline S132 degree 2 poles (23.3664, -202.8677) (24.0074, -202.8677) (24.7299, -203.5457) (24.7299, -204.1237) knots 0 0 0 1 2 2 2
  spline S133 degree 2 poles (24.7299, -204.1237) (24.7299, -204.3942) (24.6039, -204.8462) (24.4927, -205.0389) knots 0 0 0 1 2 2 2
  spline S134 degree 2 poles (24.4927, -205.0389) (24.3816, -205.2389) (24.0593, -205.6317) (23.8814, -205.8206) knots 0 0 0 1 2 2 2
  spline S135 degree 2 poles (23.8814, -205.8206) (23.5924, -206.1355) (22.8848, -206.8099) (22.6736, -207.0062) knots 0 0 0 1 2 2 2
  line L114 (22.6736, -207.0062) -> (24.9188, -207.0062)
  line L115 (24.9188, -207.0062) -> (24.9188, -207.536)
  line L116 (27.4308, -202.7603) -> (25.6413, -208.529)
  line L117 (25.6413, -208.529) -> (25.1226, -208.529)
  line L118 (25.1226, -208.529) -> (26.9047, -202.7603)
  line L119 (26.9047, -202.7603) -> (27.4308, -202.7603)
  line L120 (30.7542, -207.536) -> (27.9347, -207.536)
  line L121 (27.9347, -207.536) -> (27.9347, -206.8877)
  spline S136 degree 2 poles (27.9347, -206.8877) (28.2385, -206.6024) (28.7795, -206.0726) (29.0388, -205.7873) knots 0 0 0 1 2 2 2
  spline S137 degree 2 poles (29.0388, -205.7873) (29.5612, -205.213) (29.9428, -204.5239) (29.9428, -204.1571) knots 0 0 0 1 2 2 2
  spline S138 degree 2 poles (29.9428, -204.1571) (29.9428, -203.9644) (29.8243, -203.6754) (29.7168, -203.5828) knots 0 0 0 1 2 2 2
  spline S139 degree 2 poles (29.7168, -203.5828) (29.6094, -203.4902) (29.3278, -203.3975) (29.1574, -203.3975) knots 0 0 0 1 2 2 2
  spline S140 degree 2 poles (29.1574, -203.3975) (28.9943, -203.3975) (28.6609, -203.479) (28.509, -203.542) knots 0 0 0 1 2 2 2
  spline S141 degree 2 poles (28.509, -203.542) (28.3793, -203.5939) (28.1385, -203.7421) (28.0644, -203.794) knots 0 0 0 1 2 2 2
  line L122 (28.0644, -203.794) -> (28.031, -203.794)
  line L123 (28.031, -203.794) -> (28.031, -203.1419)
  spline S142 degree 2 poles (28.031, -203.1419) (28.22, -203.0493) (28.898, -202.8677) (29.2018, -202.8677) knots 0 0 0 1 2 2 2
  spline S143 degree 2 poles (29.2018, -202.8677) (29.8428, -202.8677) (30.5653, -203.5457) (30.5653, -204.1237) knots 0 0 0 1 2 2 2
  spline S144 degree 2 poles (30.5653, -204.1237) (30.5653, -204.3942) (30.4393, -204.8462) (30.3282, -205.0389) knots 0 0 0 1 2 2 2
  spline S145 degree 2 poles (30.3282, -205.0389) (30.217, -205.2389) (29.8947, -205.6317) (29.7168, -205.8206) knots 0 0 0 1 2 2 2
  spline S146 degree 2 poles (29.7168, -205.8206) (29.4278, -206.1355) (28.7202, -206.8099) (28.509, -207.0062) knots 0 0 0 1 2 2 2
  line L124 (28.509, -207.0062) -> (30.7542, -207.0062)
  line L125 (30.7542, -207.0062) -> (30.7542, -207.536)
  spline S147 degree 2 poles (34.211, -205.25) (34.211, -206.4801) (33.496, -207.6324) (32.7512, -207.6324) knots 0 0 0 1 2 2 2
  spline S148 degree 2 poles (32.7512, -207.6324) (31.9954, -207.6324) (31.2878, -206.4579) (31.2878, -205.2537) knots 0 0 0 1 2 2 2
  spline S149 degree 2 poles (31.2878, -205.2537) (31.2878, -204.0163) (32.0028, -202.8714) (32.7512, -202.8714) knots 0 0 0 1 2 2 2
  spline S150 degree 2 poles (32.7512, -202.8714) (33.5034, -202.8714) (34.211, -204.057) (34.211, -205.25) knots 0 0 0 1 2 2 2
  spline S151 degree 2 poles (33.4256, -206.6431) (33.5145, -206.4171) (33.5886, -205.7206) (33.5886, -205.25) knots 0 0 0 1 2 2 2
  spline S152 degree 2 poles (33.5886, -205.25) (33.5886, -204.7795) (33.5145, -204.0867) (33.4219, -203.8532) knots 0 0 0 1 2 2 2
  spline S153 degree 2 poles (33.4219, -203.8532) (33.3292, -203.6198) (33.0069, -203.379) (32.7512, -203.379) knots 0 0 0 1 2 2 2
  spline S154 degree 2 poles (32.7512, -203.379) (32.4956, -203.379) (32.1658, -203.6198) (32.0695, -203.8607) knots 0 0 0 1 2 2 2
  spline S155 degree 2 poles (32.0695, -203.8607) (31.9769, -204.0941) (31.9102, -204.8054) (31.9102, -205.2537) knots 0 0 0 1 2 2 2
  spline S156 degree 2 poles (31.9102, -205.2537) (31.9102, -205.7354) (31.9695, -206.3801) (32.0658, -206.632) knots 0 0 0 1 2 2 2
  spline S157 degree 2 poles (32.0658, -206.632) (32.1547, -206.8691) (32.4845, -207.1248) (32.7512, -207.1248) knots 0 0 0 1 2 2 2
  spline S158 degree 2 poles (32.7512, -207.1248) (33.0032, -207.1248) (33.3329, -206.884) (33.4256, -206.6431) knots 0 0 0 1 2 2 2
  line L126 (37.6159, -207.536) -> (34.7964, -207.536)
  line L127 (34.7964, -207.536) -> (34.7964, -206.8877)
  spline S159 degree 2 poles (34.7964, -206.8877) (35.1002, -206.6024) (35.6412, -206.0726) (35.9005, -205.7873) knots 0 0 0 1 2 2 2
  spline S160 degree 2 poles (35.9005, -205.7873) (36.4229, -205.213) (36.8045, -204.5239) (36.8045, -204.1571) knots 0 0 0 1 2 2 2
  spline S161 degree 2 poles (36.8045, -204.1571) (36.8045, -203.9644) (36.686, -203.6754) (36.5785, -203.5828) knots 0 0 0 1 2 2 2
  spline S162 degree 2 poles (36.5785, -203.5828) (36.4711, -203.4902) (36.1895, -203.3975) (36.0191, -203.3975) knots 0 0 0 1 2 2 2
  spline S163 degree 2 poles (36.0191, -203.3975) (35.8561, -203.3975) (35.5226, -203.479) (35.3707, -203.542) knots 0 0 0 1 2 2 2
  spline S164 degree 2 poles (35.3707, -203.542) (35.241, -203.5939) (35.0002, -203.7421) (34.9261, -203.794) knots 0 0 0 1 2 2 2
  line L128 (34.9261, -203.794) -> (34.8927, -203.794)
  line L129 (34.8927, -203.794) -> (34.8927, -203.1419)
  spline S165 degree 2 poles (34.8927, -203.1419) (35.0817, -203.0493) (35.7597, -202.8677) (36.0635, -202.8677) knots 0 0 0 1 2 2 2
  spline S166 degree 2 poles (36.0635, -202.8677) (36.7045, -202.8677) (37.427, -203.5457) (37.427, -204.1237) knots 0 0 0 1 2 2 2
  spline S167 degree 2 poles (37.427, -204.1237) (37.427, -204.3942) (37.301, -204.8462) (37.1899, -205.0389) knots 0 0 0 1 2 2 2
  spline S168 degree 2 poles (37.1899, -205.0389) (37.0787, -205.2389) (36.7564, -205.6317) (36.5785, -205.8206) knots 0 0 0 1 2 2 2
  spline S169 degree 2 poles (36.5785, -205.8206) (36.2895, -206.1355) (35.5819, -206.8099) (35.3707, -207.0062) knots 0 0 0 1 2 2 2
  line L130 (35.3707, -207.0062) -> (37.6159, -207.0062)
  line L131 (37.6159, -207.0062) -> (37.6159, -207.536)
  spline S170 degree 2 poles (41.1172, -206.054) (41.1172, -206.406) (40.8838, -207.0025) (40.6874, -207.2026) knots 0 0 0 1 2 2 2
  spline S171 degree 2 poles (40.6874, -207.2026) (40.4836, -207.4138) (39.9723, -207.6324) (39.6648, -207.6324) knots 0 0 0 1 2 2 2
  spline S172 degree 2 poles (39.6648, -207.6324) (39.3573, -207.6324) (38.8497, -207.4249) (38.6571, -207.2174) knots 0 0 0 1 2 2 2
  spline S173 degree 2 poles (38.6571, -207.2174) (38.4199, -206.9692) (38.1532, -206.1355) (38.1532, -205.5279) knots 0 0 0 1 2 2 2
  spline S174 degree 2 poles (38.1532, -205.5279) (38.1532, -204.9314) (38.3977, -203.9718) (38.6533, -203.6161) knots 0 0 0 1 2 2 2
  spline S175 degree 2 poles (38.6533, -203.6161) (38.9016, -203.2679) (39.687, -202.8788) (40.202, -202.8788) knots 0 0 0 1 2 2 2
  spline S176 degree 2 poles (40.202, -202.8788) (40.354, -202.8788) (40.6207, -202.9085) (40.7208, -202.9418) knots 0 0 0 1 2 2 2
  line L132 (40.7208, -202.9418) -> (40.7208, -203.5309)
  line L133 (40.7208, -203.5309) -> (40.6948, -203.5309)
  spline S177 degree 2 poles (40.6948, -203.5309) (40.6096, -203.4865) (40.2984, -203.4086) (40.1205, -203.4086) knots 0 0 0 1 2 2 2
  spline S178 degree 2 poles (40.1205, -203.4086) (39.55, -203.4086) (38.8497, -204.1793) (38.783, -204.9351) knots 0 0 0 1 2 2 2
  spline S179 degree 2 poles (38.783, -204.9351) (39.0016, -204.7832) (39.461, -204.6165) (39.7352, -204.6165) knots 0 0 0 1 2 2 2
  spline S180 degree 2 poles (39.7352, -204.6165) (40.002, -204.6165) (40.4021, -204.7239) (40.6207, -204.887) knots 0 0 0 1 2 2 2
  spline S181 degree 2 poles (40.6207, -204.887) (40.8727, -205.0759) (41.1172, -205.6613) (41.1172, -206.054) knots 0 0 0 1 2 2 2
  spline S182 degree 2 poles (40.4947, -206.08) (40.4947, -205.7984) (40.3465, -205.4168) (40.1835, -205.2834) knots 0 0 0 1 2 2 2
  spline S183 degree 2 poles (40.1835, -205.2834) (40.0613, -205.1871) (39.7574, -205.1241) (39.5981, -205.1241) knots 0 0 0 1 2 2 2
  spline S184 degree 2 poles (39.5981, -205.1241) (39.3832, -205.1241) (38.9794, -205.2537) (38.783, -205.376) knots 0 0 0 1 2 2 2
  spline S185 degree 2 poles (38.783, -205.376) (38.7793, -205.4427) (38.7719, -205.5687) (38.7719, -205.665) knots 0 0 0 1 2 2 2
  spline S186 degree 2 poles (38.7719, -205.665) (38.7719, -206.1392) (38.9572, -206.7209) (39.0979, -206.8728) knots 0 0 0 1 2 2 2
  spline S187 degree 2 poles (39.0979, -206.8728) (39.2276, -207.0173) (39.5092, -207.1322) (39.6685, -207.1322) knots 0 0 0 1 2 2 2
  spline S188 degree 2 poles (39.6685, -207.1322) (40.039, -207.1322) (40.4947, -206.6061) (40.4947, -206.08) knots 0 0 0 1 2 2 2
  point P0 (0, 0)
  constraints: 2 other
emboss "Emboss1" sketch "Sketch13" operation cut depth 2.54 direction (-1, 0, 0)